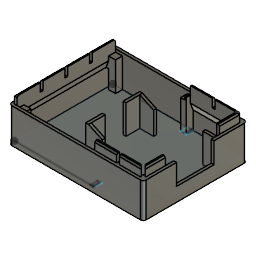
MorseDeck Terminal Bottom Shell (Autodesk Fusion 360 design; units mm, degrees)
part number: 2026-05-24-20-41-13-399
Autodesk Fusion 360 part; units mm, degrees
sketch "Sketch1" plane through (0, 0, 0) normal (0, 0, 1) x (1, 0, 0)
  line L0 (0, 0) -> (97, 0)
  line L1 (97, 0) -> (97, 75)
  line L2 (97, 75) -> (0, 75)
  line L3 (0, 75) -> (0, 0)
  dimension "d1" = 97
  dimension "d2" = 75
  constraint horizontal L0
  constraint vertical L1
  constraint horizontal L2
  constraint vertical L3
  constraint coincident L0.start L3.end
  measures "d1" distance of L0.start L0.end
  measures "d2" distance of L0.start L2.end
extrude "Extrude1" add sketch "Sketch1" along normal blind 24
shell "Shell1" thickness 2 removed faces 1 at (32.3333, 25, 24)
sketch "Sketch2" plane through (97, 0, 0) normal (1, 0, 0) x (0, 1, 0)
  line L0 (0, 0) -> (75, 0)
  line L1 (75, 0) -> (75, 24)
  line L2 (75, 24) -> (0, 24)
  line L3 (0, 24) -> (0, 0)
  line L4 (37.5, 24) -> (24, 24)
  line L5 (24, 24) -> (24, 10)
  line L6 (24, 10) -> (37.5, 10)
  line L7 (37.5, 10) -> (37.5, 24)
  line L8 (37.5, 24) -> (51, 24)
  line L9 (51, 24) -> (51, 10)
  line L10 (51, 10) -> (37.5, 10)
  line L11 (37.5, 10) -> (37.5, 24)
  dimension "d6" = 13.5
  dimension "d7" = 14
  constraint horizontal L4
  constraint vertical L5
  constraint horizontal L6
  constraint vertical L7
  constraint midpoint L2 L4.start
  constraint horizontal L8
  constraint vertical L9
  constraint horizontal L10
  constraint vertical L11
  measures "d6" distance of L4.start L4.end
  measures "d7" distance of L4.start L6.end
extrude "Extrude2" cut sketch "Sketch2" against normal blind 12 contours L2 L4 L5 L6 L7 L11 | L2 L7 L8 L9 L10 L11
sketch "Sketch3" plane through (0, 0, 2) normal (0, 0, 1) x (-1, 0, 0)
  line L0 (-2, -73) -> (-2, -2)
  line L1 (-2, -2) -> (-95, -2)
  line L2 (-95, -2) -> (-95, -73)
  line L3 (-95, -73) -> (-2, -73)
  line L4 (-95, -37.5) -> (-95, -20)
  line L5 (-95, -37.5) -> (-95, -55)
  line L6 (-95, -20) -> (-39.5, -20)
  line L7 (-39.5, -20) -> (-39.5, -55)
  line L8 (-39.5, -55) -> (-95, -55)
  line L9 (-39.5, -55) -> (-37.5, -55)
  line L10 (-37.5, -55) -> (-37.5, -45)
  line L11 (-37.5, -45) -> (-39.5, -45)
  line L12 (-39.5, -45) -> (-39.5, -55)
  line L13 (-37.5, -55) -> (-49.5, -55)
  line L14 (-49.5, -55) -> (-49.5, -57)
  line L15 (-49.5, -57) -> (-37.5, -57)
  line L16 (-37.5, -57) -> (-37.5, -55)
  line L17 (-39.5, -20) -> (-37.5, -20)
  line L18 (-37.5, -20) -> (-37.5, -30)
  line L19 (-37.5, -30) -> (-39.5, -30)
  line L20 (-39.5, -30) -> (-39.5, -20)
  line L21 (-37.5, -20) -> (-49.5, -20)
  line L22 (-49.5, -20) -> (-49.5, -18)
  line L23 (-49.5, -18) -> (-37.5, -18)
  line L24 (-37.5, -18) -> (-37.5, -20)
  line L25 (-95, -55) -> (-85, -55)
  line L26 (-85, -55) -> (-85, -57)
  line L27 (-85, -57) -> (-95, -57)
  line L28 (-95, -57) -> (-95, -55)
  line L29 (-95, -20) -> (-85, -20)
  line L30 (-85, -20) -> (-85, -18)
  line L31 (-85, -18) -> (-95, -18)
  line L32 (-95, -18) -> (-95, -20)
  dimension "d10" = 17.5
  dimension "d11" = 17.5
  dimension "d12" = 55.5
  dimension "d13" = 35
  dimension "d14" = 2
  dimension "d15" = 12
  dimension "d16" = 2
  dimension "d17" = 2
  dimension "d18" = 10
  dimension "d19" = 12
  dimension "d20" = 10
  dimension "d21" = 2
  dimension "d22" = 10
  constraint midpoint L2 L4.start
  constraint perpendicular L1 L4
  constraint perpendicular L1 L5
  constraint perpendicular L4 L6
  constraint perpendicular L6 L7
  constraint horizontal L9
  constraint vertical L10
  constraint horizontal L11
  constraint vertical L12
  constraint horizontal L13
  constraint vertical L14
  constraint horizontal L15
  constraint vertical L16
  constraint horizontal L17
  constraint vertical L18
  constraint horizontal L19
  constraint vertical L20
  constraint horizontal L21
  constraint vertical L22
  constraint horizontal L23
  constraint vertical L24
  constraint horizontal L25
  constraint vertical L26
  constraint horizontal L27
  constraint vertical L28
  constraint horizontal L29
  constraint vertical L30
  constraint horizontal L31
  constraint vertical L32
  measures "d10" distance of L4.start L4.end
  measures "d11" distance of L4.start L5.end
  measures "d12" distance of L4.end L6.end
  measures "d13" distance of L6.end L7.end
  measures "d14" distance of L7.end L9.end
  measures "d15" distance of L9.end L13.end
  measures "d16" distance of L9.end L15.end
  measures "d17" distance of L6.end L17.end
  measures "d18" distance of L6.end L19.end
  measures "d19" distance of L17.end L21.end
  measures "d20" distance of L5.end L25.end
  measures "d21" distance of L5.end L27.end
  measures "d22" distance of L4.end L29.end
extrude "Extrude3" add sketch "Sketch3" along normal blind 21 contours L2 L8 L25 L26 L27 L28 | L2 L6 L29 L30 L31 L32 | L8 L9 L13 L14 L15 L16 | L6 L17 L21 L22 L23 L24 | L7 L9 L10 L11 L12 L13 | L7 L17 L18 L19 L20 L21
sketch "Sketch4" plane through (0, 0, 2) normal (0, 0, 1) x (-1, 0, 0)
  line L0 (-85, -20) -> (-95, -20)
  line L1 (-95, -20) -> (-95, -55)
  line L2 (-95, -55) -> (-85, -55)
  line L3 (-85, -55) -> (-85, -57)
  line L4 (-85, -57) -> (-95, -57)
  line L5 (-95, -57) -> (-95, -73)
  line L6 (-95, -73) -> (-2, -73)
  line L7 (-2, -73) -> (-2, -2)
  line L8 (-2, -2) -> (-95, -2)
  line L9 (-95, -2) -> (-95, -18)
  line L10 (-95, -18) -> (-85, -18)
  line L11 (-85, -18) -> (-85, -20)
  line L12 (-37.5, -18) -> (-37.5, -30)
  line L13 (-37.5, -30) -> (-39.5, -30)
  line L14 (-39.5, -30) -> (-39.5, -20)
  line L15 (-39.5, -20) -> (-49.5, -20)
  line L16 (-49.5, -20) -> (-49.5, -18)
  line L17 (-49.5, -18) -> (-37.5, -18)
  line L18 (-37.5, -57) -> (-49.5, -57)
  line L19 (-49.5, -57) -> (-49.5, -55)
  line L20 (-49.5, -55) -> (-39.5, -55)
  line L21 (-39.5, -55) -> (-39.5, -45)
  line L22 (-39.5, -45) -> (-37.5, -45)
  line L23 (-37.5, -45) -> (-37.5, -57)
  line L24 (-2, -2) -> (-59, -2)
  line L25 (-59, -2) -> (-57, -2)
  line L26 (-57, -2) -> (-57, -7)
  line L27 (-57, -7) -> (-59, -7)
  line L28 (-59, -7) -> (-59, -2)
  line L29 (-59, -2) -> (-60, -2)
  line L30 (-60, -2) -> (-60, -7)
  line L31 (-60, -7) -> (-59, -7)
  line L32 (-59, -7) -> (-59, -2)
  line L33 (-2, -73) -> (-59, -73)
  line L34 (-59, -73) -> (-56, -73)
  line L35 (-56, -73) -> (-56, -68)
  line L36 (-56, -68) -> (-59, -68)
  line L37 (-59, -68) -> (-59, -73)
  line L38 (-59, -73) -> (-60, -73)
  line L39 (-60, -73) -> (-60, -68)
  line L40 (-60, -68) -> (-59, -68)
  line L41 (-59, -68) -> (-59, -73)
  dimension "d25" = 57
  dimension "d26" = 2
  dimension "d27" = 5
  dimension "d28" = 57
  constraint coincident L7.end L8.start
  constraint perpendicular L7 L24
  constraint horizontal L25
  constraint vertical L26
  constraint horizontal L27
  constraint vertical L28
  constraint horizontal L29
  constraint vertical L30
  constraint horizontal L31
  constraint vertical L32
  constraint coincident L6.end L7.start
  constraint perpendicular L7 L33
  constraint horizontal L34
  constraint vertical L35
  constraint horizontal L36
  constraint vertical L37
  constraint horizontal L38
  constraint vertical L39
  constraint horizontal L40
  constraint vertical L41
  measures "d25" distance of L7.end L24.end
  measures "d26" distance of L24.end L25.end
  measures "d27" distance of L24.end L27.end
  measures "d28" distance of L6.end L33.end
extrude "Extrude4" add sketch "Sketch4" along normal blind 21 contours L8 L24 L25 L26 L27 L28 L32 | L6 L33 L34 L35 L36 L37 L41
extrude "Extrude5" add sketch "Sketch4" along normal blind 23 contours L8 L28 L29 L30 L31 L32 | L6 L37 L38 L39 L40 L41
extrude "Extrude6" add 1 faces at (52, 74.3333, 24) along direction (0, 0, 1) blind 1
sketch "Sketch5" plane through (0, 0, 2) normal (0, 0, 1) x (-1, 0, 0)
  line L0 (-4, -2) -> (-9, -2)
  line L1 (-9, -2) -> (-9, -7)
  line L2 (-9, -7) -> (-4, -7)
  line L3 (-4, -7) -> (-4, -2)
  line L4 (-4, -73) -> (-9, -73)
  line L5 (-9, -73) -> (-9, -68)
  line L6 (-9, -68) -> (-4, -68)
  line L7 (-4, -68) -> (-4, -73)
  line L8 (-2, -73) -> (-2, -2)
  dimension "d35" = 5
  dimension "d36" = 5
  dimension "d37" = 5
  dimension "d38" = 5
  dimension "d69" = 2
  dimension "d70" = 2
  constraint horizontal L0
  constraint vertical L1
  constraint horizontal L2
  constraint vertical L3
  constraint horizontal L4
  constraint vertical L5
  constraint horizontal L6
  constraint vertical L7
  measures "d35" distance of L0.start L0.end
  measures "d36" distance of L0.start L2.end
  measures "d37" distance of L4.start L4.end
  measures "d38" distance of L4.start L6.end
  measures "d69" distance of L3 L8
  measures "d70" distance of L7 L8
extrude "Extrude7" add sketch "Sketch5" along normal blind 21
sketch "Sketch6" plane through (0, 73, 0) normal (0, -1, 0) x (1, 0, 0)
  line L0 (60, 25) -> (60, 2)
  line L1 (60, 2) -> (95, 2)
  line L2 (95, 2) -> (95, 25)
  line L3 (95, 25) -> (60, 25)
  line L4 (95, 25) -> (60, 25)
  line L5 (60, 25) -> (60, 15)
  line L6 (60, 15) -> (95, 15)
  line L7 (95, 15) -> (95, 25)
  dimension "d41" = 10
  constraint horizontal L4
  constraint vertical L5
  constraint horizontal L6
  constraint vertical L7
  constraint coincident L2.end L3.start
  constraint collinear L0 L5
  measures "d41" distance of L2.end L6.end
sketch "Sketch15" plane through (95, 0, 0) normal (-1, 0, 0) x (0, -1, 0)
  line L0 (-20, 2) -> (-20, 23)
  line L1 (-20, 23) -> (-18, 23)
  line L2 (-18, 23) -> (-18, 2)
  line L3 (-18, 2) -> (-2, 2)
  line L4 (-2, 2) -> (-2, 25)
  line L5 (-2, 25) -> (-24, 25)
  line L6 (-24, 25) -> (-24, 10)
  line L7 (-24, 10) -> (-51, 10)
  line L8 (-51, 10) -> (-51, 25)
  line L9 (-51, 25) -> (-73, 25)
  line L10 (-73, 25) -> (-73, 2)
  line L11 (-73, 2) -> (-57, 2)
  line L12 (-57, 2) -> (-57, 23)
  line L13 (-57, 23) -> (-55, 23)
  line L14 (-55, 23) -> (-55, 2)
  line L15 (-55, 2) -> (-20, 2)
  line L16 (-2, 25) -> (-18, 25)
  line L17 (-18, 25) -> (-18, 15)
  line L18 (-18, 15) -> (-2, 15)
  line L19 (-2, 15) -> (-2, 25)
  line L20 (-73, 25) -> (-57, 25)
  line L21 (-57, 25) -> (-57, 15)
  line L22 (-57, 15) -> (-73, 15)
  line L23 (-73, 15) -> (-73, 25)
  dimension "d80" = 10
  dimension "d81" = 10
  constraint horizontal L16
  constraint vertical L17
  constraint horizontal L18
  constraint vertical L19
  constraint coincident L4.end L5.start
  constraint horizontal L20
  constraint vertical L21
  constraint horizontal L22
  constraint vertical L23
  constraint coincident L9.end L10.start
  measures "d80" distance of L4.end L18.end
  measures "d81" distance of L9.end L22.end
sketch "Sketch16" plane through (2, 0, 0) normal (1, 0, 0) x (0, 1, 0)
  line L0 (2, 2) -> (73, 2)
  line L1 (73, 2) -> (73, 25)
  line L2 (73, 25) -> (2, 25)
  line L3 (2, 25) -> (2, 2)
  line L4 (2, 25) -> (73, 25)
  line L5 (73, 25) -> (73, 15)
  line L6 (73, 15) -> (2, 15)
  line L7 (2, 15) -> (2, 25)
  dimension "d82" = 10
  constraint horizontal L4
  constraint vertical L5
  constraint horizontal L6
  constraint vertical L7
  constraint coincident L2.end L3.start
  measures "d82" distance of L2.end L6.end
sketch "Sketch17" plane through (0, 73, 0) normal (0, -1, 0) x (1, 0, 0)
  line L0 (60, 25) -> (60, 2)
  line L1 (60, 2) -> (95, 2)
  line L2 (95, 2) -> (95, 25)
  line L3 (95, 25) -> (60, 25)
  line L4 (60, 25) -> (95, 25)
  line L5 (95, 25) -> (95, 15)
  line L6 (95, 15) -> (60, 15)
  line L7 (60, 15) -> (60, 25)
  dimension "d83" = 10
  constraint horizontal L4
  constraint vertical L5
  constraint horizontal L6
  constraint vertical L7
  constraint coincident L0.start L3.end
  measures "d83" distance of L0.start L6.end
sketch "Sketch18" plane through (0, 2, 0) normal (0, 1, 0) x (-1, 0, 0)
  line L0 (-60, 2) -> (-60, 25)
  line L1 (-60, 25) -> (-95, 25)
  line L2 (-95, 25) -> (-95, 2)
  line L3 (-95, 2) -> (-60, 2)
  line L4 (-60, 25) -> (-95, 25)
  line L5 (-95, 25) -> (-95, 15)
  line L6 (-95, 15) -> (-60, 15)
  line L7 (-60, 15) -> (-60, 25)
  constraint horizontal L4
  constraint vertical L5
  constraint horizontal L6
  constraint vertical L7
  constraint coincident L2 L5.end
  constraint coincident L0.end L1.start
extrude "Extrude18" add sketch "Sketch15" along normal blind 2 contours L2 L4 L5 L16 L17 L18 L19 | L9 L10 L12 L20 L21 L22 L23
extrude "Extrude19" add sketch "Sketch17" along normal blind 2 contours L0 L2 L3 L4 L5 L6 L7
extrude "Extrude20" add sketch "Sketch18" along normal blind 2 contours L0 L1 L2 L4 L5 L6 L7
extrude "Extrude21" add sketch "Sketch16" along normal blind 2 contours L1 L2 L3 L4 L5 L6 L7
chamfer "Chamfer5" distance 5 angle 20 5 edges at (93, 64, 15) (76.5, 71, 15) (93, 11, 15) (76.5, 4, 15) (4, 37.5, 15) measured on face at (93, 66.3333, 21) measured on face at (71, 71, 21.6667) measured on face at (93, 8.6667, 21) measured on face at (71, 4, 18.3333) measured on face at (4, 27.3333, 20.3333)
sketch "Sketch19" plane through (0, 0, 25) normal (0, 0, 1) x (-1, 0, 0)
  line L0 (-60, -4) -> (-60, -7)
  line L1 (-60, -7) -> (-59, -7)
  line L2 (-59, -7) -> (-59, -2)
  line L3 (-59, -2) -> (-4, -2)
  line L4 (-4, -2) -> (-4, -73)
  line L5 (-4, -73) -> (-59, -73)
  line L6 (-59, -73) -> (-59, -68)
  line L7 (-59, -68) -> (-60, -68)
  line L8 (-60, -68) -> (-60, -71)
  line L9 (-60, -71) -> (-93, -71)
  line L10 (-93, -71) -> (-93, -57)
  line L11 (-93, -57) -> (-95, -57)
  line L12 (-95, -57) -> (-95, -51)
  line L13 (-95, -51) -> (-97, -51)
  line L14 (-97, -51) -> (-97, -75)
  line L15 (-97, -75) -> (0, -75)
  line L16 (0, -75) -> (0, 0)
  line L17 (0, 0) -> (-97, 0)
  line L18 (-97, 0) -> (-97, -24)
  line L19 (-97, -24) -> (-95, -24)
  line L20 (-95, -24) -> (-95, -18)
  line L21 (-95, -18) -> (-93, -18)
  line L22 (-93, -18) -> (-93, -4)
  line L23 (-93, -4) -> (-60, -4)
  line L24 (-4, -73) -> (-2, -73)
  line L25 (-2, -73) -> (-2, -2)
  line L26 (-2, -2) -> (-4, -2)
  line L27 (-4, -2) -> (-4, -73)
  line L28 (-95, -57) -> (-93, -57)
  line L29 (-93, -57) -> (-93, -71)
  line L30 (-93, -71) -> (-95, -71)
  line L31 (-95, -71) -> (-95, -57)
  line L32 (-95, -18) -> (-93, -18)
  line L33 (-93, -18) -> (-93, -4)
  line L34 (-93, -4) -> (-95, -4)
  line L35 (-95, -4) -> (-95, -18)
  line L36 (-60, -71) -> (-95, -71)
  line L37 (-95, -71) -> (-95, -73)
  line L38 (-95, -73) -> (-60, -73)
  line L39 (-60, -73) -> (-60, -71)
  line L40 (-95, -4) -> (-60, -4)
  line L41 (-60, -4) -> (-60, -2)
  line L42 (-60, -2) -> (-95, -2)
  line L43 (-95, -2) -> (-95, -4)
  dimension "d94" = 2
  constraint horizontal L24
  constraint vertical L25
  constraint horizontal L26
  constraint vertical L27
  constraint coincident L4.end L5.start
  constraint horizontal L28
  constraint vertical L29
  constraint horizontal L30
  constraint vertical L31
  constraint coincident L9.end L10.start
  constraint coincident L11.end L12.start
  constraint horizontal L32
  constraint vertical L33
  constraint horizontal L34
  constraint vertical L35
  constraint coincident L22.end L23.start
  constraint coincident L20.end L21.start
  constraint horizontal L36
  constraint vertical L37
  constraint horizontal L38
  constraint vertical L39
  constraint coincident L8.end L9.start
  constraint horizontal L40
  constraint vertical L41
  constraint horizontal L42
  constraint vertical L43
  measures "d94" distance of L4.end L24.end
extrude "Extrude22" add sketch "Sketch19" along normal blind 6 contours L23 L34 L40 L41 L42 L43 | L21 L22 L32 L33 L34 L35 L40 | L4 L24 L25 L26 L27 | L9 L30 L36 L37 L38 L39 | L10 L11 L28 L29 L30 L31 L36
sketch "Sketch21" plane through (0, 0, 31) normal (0, 0, 1) x (-1, 0, 0)
  line L0 (-95, -2) -> (-95, -18)
  line L1 (-95, -18) -> (-93, -18)
  line L2 (-93, -18) -> (-93, -4)
  line L3 (-93, -4) -> (-60, -4)
  line L4 (-60, -4) -> (-60, -2)
  line L5 (-60, -2) -> (-95, -2)
  line L6 (-93, -4) -> (-95, -2) construction
  line L7 (-93, -5.4142) -> (-95, -3.4142)
  line L8 (-91.5858, -4) -> (-93.5858, -2)
  dimension "d99" = 1
  dimension "d100" = 1
  constraint coincident L2.end L3.start
  constraint coincident L0.start L5.end
  constraint coincident L2 L7.start
  constraint coincident L0 L7.end
  constraint coincident L3 L8.start
  constraint coincident L5 L8.end
  constraint parallel L6 L7
  constraint parallel L6 L8
  measures "d99" distance of L6 L7
  measures "d100" distance of L6 L8
extrude "Extrude23" cut sketch "Sketch21" against normal blind 6 contours L0 L2 L3 L5 L7 L8
sketch "Sketch22" plane through (0, 0, 31) normal (0, 0, 1) x (-1, 0, 0)
  line L0 (-95, -57) -> (-95, -73)
  line L1 (-95, -73) -> (-60, -73)
  line L2 (-60, -73) -> (-60, -71)
  line L3 (-60, -71) -> (-93, -71)
  line L4 (-93, -71) -> (-93, -57)
  line L5 (-93, -57) -> (-95, -57)
  line L6 (-95, -73) -> (-93, -71) construction
  line L7 (-93.5858, -73) -> (-91.5858, -71)
  line L8 (-95, -71.5858) -> (-93, -69.5858)
  dimension "d103" = 1
  dimension "d104" = 1
  constraint coincident L0.end L1.start
  constraint coincident L3.end L4.start
  constraint coincident L1 L7.start
  constraint coincident L3 L7.end
  constraint coincident L0 L8.start
  constraint coincident L4 L8.end
  constraint parallel L7 L8
  constraint parallel L6 L7
  measures "d103" distance of L6 L7
  measures "d104" distance of L6 L8
extrude "Extrude24" cut sketch "Sketch22" against normal blind 6 contours L0 L1 L3 L4 L7 L8
sketch "Sketch23" plane through (2, 0, 0) normal (-1, 0, 0) x (0, -1, 0)
  line L0 (-73, 25) -> (-2, 25)
  line L1 (-2, 25) -> (-2, 31)
  line L2 (-2, 31) -> (-73, 31)
  line L3 (-73, 31) -> (-73, 25)
  line L4 (-37.5, 31) -> (-37.5, 25) construction
  line L5 (-55.25, 31) -> (-55.25, 25) construction
  line L6 (-19.75, 31) -> (-19.75, 25) construction
  line L7 (-54.25, 31) -> (-56.25, 31)
  line L8 (-56.25, 31) -> (-56.25, 25)
  line L9 (-56.25, 25) -> (-54.25, 25)
  line L10 (-54.25, 25) -> (-54.25, 31)
  line L11 (-54.25, 31) -> (-56.25, 25) construction
  line L12 (-56.25, 31) -> (-54.25, 25) construction
  line L13 (-36.5, 31) -> (-38.5, 31)
  line L14 (-38.5, 31) -> (-38.5, 25)
  line L15 (-38.5, 25) -> (-36.5, 25)
  line L16 (-36.5, 25) -> (-36.5, 31)
  line L17 (-36.5, 31) -> (-38.5, 25) construction
  line L18 (-38.5, 31) -> (-36.5, 25) construction
  line L19 (-18.75, 31) -> (-20.75, 31)
  line L20 (-20.75, 31) -> (-20.75, 25)
  line L21 (-20.75, 25) -> (-18.75, 25)
  line L22 (-18.75, 25) -> (-18.75, 31)
  line L23 (-18.75, 31) -> (-20.75, 25) construction
  line L24 (-20.75, 31) -> (-18.75, 25) construction
  point P0 (-55.25, 28)
  point P1 (-37.5, 28)
  point P2 (-19.75, 28)
  dimension "d109" = 17.75
  dimension "d110" = 17.75
  dimension "d111" = 2
  dimension "d112" = 2
  dimension "d113" = 2
  dimension "d114" = 6
  constraint midpoint L2 L4.start
  constraint midpoint L0 L4.end
  constraint coincident L2 L5.start
  constraint coincident L0 L5.end
  constraint perpendicular L0 L5
  constraint coincident L2 L6.start
  constraint coincident L0 L6.end
  constraint perpendicular L0 L6
  constraint horizontal L7
  constraint perpendicular L7 L8
  constraint parallel L7 L9
  constraint parallel L8 L10
  constraint coincident L11 P0
  constraint coincident L12 P0
  constraint midpoint L5 P0
  constraint horizontal L13
  constraint perpendicular L13 L14
  constraint parallel L13 L15
  constraint parallel L14 L16
  constraint coincident L17 P1
  constraint coincident L18 P1
  constraint midpoint L4 P1
  constraint horizontal L19
  constraint perpendicular L19 L20
  constraint parallel L19 L21
  constraint parallel L20 L22
  constraint coincident L23 P2
  constraint coincident L24 P2
  constraint midpoint L6 P2
  measures "d109" distance of L3 L5
  measures "d110" distance of L1 L6
  measures "d111" distance of L8.end L9.end
  measures "d112" distance of L14.end L15.end
  measures "d113" distance of L20.end L21.end
  measures "d114" distance of L19.end L20.end
extrude "Extrude25" cut sketch "Sketch23" against normal blind 2 contours L0 L2 L7 L8 L9 L10 | L0 L2 L13 L14 L15 L16 | L0 L2 L19 L20 L21 L22
sketch "Sketch24" plane through (0, 2, 0) normal (0, -1, 0) x (1, 0, 0)
  line L0 (93.5858, 25) -> (93.5858, 31)
  line L1 (93.5858, 31) -> (60, 31)
  line L2 (60, 31) -> (60, 25)
  line L3 (60, 25) -> (93.5858, 25)
  line L4 (76.7929, 31) -> (76.7929, 25) construction
  line L5 (77.7929, 31) -> (75.7929, 31)
  line L6 (75.7929, 31) -> (75.7929, 25)
  line L7 (75.7929, 25) -> (77.7929, 25)
  line L8 (77.7929, 25) -> (77.7929, 31)
  line L9 (77.7929, 31) -> (75.7929, 25) construction
  line L10 (75.7929, 31) -> (77.7929, 25) construction
  point P0 (76.7929, 28)
  dimension "d117" = 2
  constraint midpoint L1 L4.start
  constraint midpoint L3 L4.end
  constraint horizontal L5
  constraint perpendicular L5 L6
  constraint parallel L5 L7
  constraint parallel L6 L8
  constraint coincident L9 P0
  constraint coincident L10 P0
  constraint midpoint L4 P0
  measures "d117" distance of L6.end L7.end
extrude "Extrude26" cut sketch "Sketch24" against normal blind 2 contours L1 L3 L5 L6 L7 L8
sketch "Sketch25" plane through (0, 73, 0) normal (0, 1, 0) x (-1, 0, 0)
  line L0 (-93.5858, 31) -> (-93.5858, 25)
  line L1 (-93.5858, 25) -> (-60, 25)
  line L2 (-60, 25) -> (-60, 31)
  line L3 (-60, 31) -> (-93.5858, 31)
  line L4 (-76.7929, 31) -> (-76.7929, 25) construction
  line L5 (-75.7929, 31) -> (-77.7929, 31)
  line L6 (-77.7929, 31) -> (-77.7929, 25)
  line L7 (-77.7929, 25) -> (-75.7929, 25)
  line L8 (-75.7929, 25) -> (-75.7929, 31)
  line L9 (-75.7929, 31) -> (-77.7929, 25) construction
  line L10 (-77.7929, 31) -> (-75.7929, 25) construction
  point P0 (-76.7929, 28)
  dimension "d120" = 2
  constraint midpoint L3 L4.start
  constraint midpoint L1 L4.end
  constraint horizontal L5
  constraint perpendicular L5 L6
  constraint parallel L5 L7
  constraint parallel L6 L8
  constraint coincident L9 P0
  constraint coincident L10 P0
  constraint midpoint L4 P0
  measures "d120" distance of L6.end L7.end
extrude "Extrude27" cut sketch "Sketch25" against normal blind 2 contours L1 L3 L5 L6 L7 L8
chamfer "Chamfer6" distance 1 angle 45 12 edges at (2, 64.625, 31) (2, 46.375, 31) (2, 28.625, 31) (2, 10.375, 31) (3, 2, 31) (3, 73, 31) (85.6893, 73, 31) (67.8964, 73, 31) (95, 64.2929, 31) (95, 10.7071, 31) (67.8964, 2, 31) (85.6893, 2, 31) measured on face at (2.6667, 67.4167, 31) measured on face at (3.3333, 43.75, 31) measured on face at (3.3333, 26, 31) measured on face at (3.3333, 13.1667, 31) measured on face at (3.3333, 13.1667, 31) measured on face at (2.6667, 67.4167, 31) measured on face at (87.6548, 72.3333, 31) measured on face at (65.2643, 72.3333, 31) measured on face at (94.3333, 65.8619, 31) measured on face at (94.3333, 8.9428, 31) measured on face at (70.5286, 2.6667, 31) measured on face at (87.6548, 2.6667, 31)
chamfer "Chamfer7" distance 10 angle 25 2 edges at (49.5, 19, 23) (49.5, 56, 23) measured on face at (38.1667, 22.6667, 23) measured on face at (42.1667, 56.3333, 23)
fillet "Fillet2" radius 2 4 edges at (0, 0, 12.5) (0, 75, 12.5) (97, 75, 12.5) (97, 0, 12.5)
